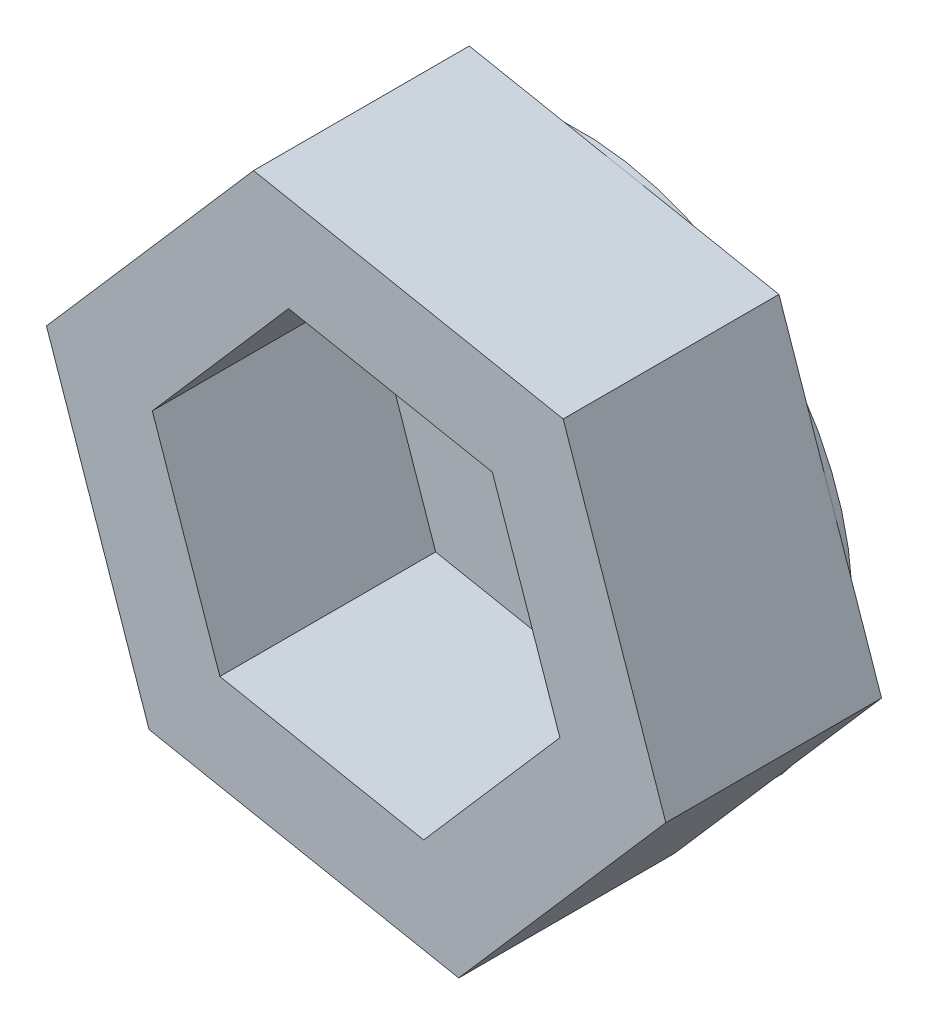
# Autodesk Inventor part: Part1
Saved by Autodesk Inventor 2014 SP1 (Build 180222100, 222)
## iProperties
Created: 2014-01-09
Part Number: Part1
Material: Generic
Document SubType Name: Modeling
Designer: Arpan
Density: 1 g/cm^3
Appearance: Default
Mass: 1.45957 g
Surface Area: 14.531 cm^2
Volume: 1.45957 cm^3
Author: Arpan
Autodesk Inventor part; units mm, degrees
ref_plane "YZ Plane" through (0, 0, 0) normal (1, 0, 0) x (0, 1, 0)
ref_plane "XZ Plane" through (0, 0, 0) normal (0, 1, 0) x (-1, 0, 0)
ref_plane "XY Plane" through (0, 0, 0) normal (0, 0, 1) x (1, 0, 0)
ref_plane "Work Plane1" through (500.3579, 35.9816, 443.1665) normal (0, 0, -1) x (0.6678, 0.7444, 0)
sketch "Sketch2" plane through (500.3579, 35.9816, 443.1665) normal (0, 0, -1) x (0.6678, 0.7444, 0)
  line L0 (3.7629, 6.2932) -> (-3.5686, 6.4054) projected
  line L1 (-3.5686, 6.4054) -> (-7.3315, 0.1122) projected
  line L2 (-7.3315, 0.1122) -> (-3.7629, -6.2932) projected
  line L3 (-3.7629, -6.2932) -> (3.5686, -6.4054) projected
  line L4 (3.5686, -6.4054) -> (7.3315, -0.1122) projected
  line L5 (7.3315, -0.1122) -> (3.7629, 6.2932) projected
  line L6 (-7.3315, 0.1122) -> (7.3315, -0.1122)
  line L7 (3.7629, 6.2932) -> (-3.7629, -6.2932)
  line L8 (-3.5686, 6.4054) -> (3.5686, -6.4054)
  line L9 (-3.5686, 6.4054) -> (-5.4229, 9.7337)
  line L10 (-5.4229, 9.7337) -> (5.7182, 9.5632)
  line L11 (5.7182, 9.5632) -> (11.141, -0.1705)
  line L12 (11.141, -0.1705) -> (5.4229, -9.7337)
  line L13 (5.4229, -9.7337) -> (-5.7182, -9.5632)
  line L14 (-5.7182, -9.5632) -> (-11.141, 0.1705)
  line L15 (-11.141, 0.1705) -> (-5.4229, 9.7337)
  point P0 (-360.9105, -348.4198)
  point P1 (0, 0)
  dimension "d0" = 3.81
  constraints: 20 end point, 3 parallel, 1 collinear, 1 midpoint, 13 other
  measures "d0" distance of L0.end L9.end
extrude "Extrusion1" add sketch "Sketch2" against normal blind 7.62
sketch "Sketch3" plane through (500.3579, 35.9816, 443.1665) normal (0, 0, -1) x (-0.7444, 0.6678, 0)
  line L0 (-6.2932, 3.7629) -> (0.1122, 7.3315) projected
  line L1 (0.1122, 7.3315) -> (6.4054, 3.5686) projected
  line L2 (6.4054, 3.5686) -> (6.2932, -3.7629) projected
  line L3 (6.2932, -3.7629) -> (-0.1122, -7.3315) projected
  line L4 (-0.1122, -7.3315) -> (-6.4054, -3.5686) projected
  line L5 (-6.4054, -3.5686) -> (-6.2932, 3.7629) projected
  line L6 (-9.7337, -5.4229) -> (-0.1705, -11.141) projected
  line L7 (-0.1705, -11.141) -> (9.5632, -5.7182) projected
  line L8 (9.5632, -5.7182) -> (9.7337, 5.4229) projected
  line L9 (9.7337, 5.4229) -> (0.1705, 11.141) projected
  line L10 (0.1705, 11.141) -> (-9.5632, 5.7182) projected
  line L11 (-9.5632, 5.7182) -> (-9.7337, -5.4229) projected
  point P0 (348.4198, -360.9105)
sketch "Sketch4" plane through (500.3579, 35.9816, 443.1665) normal (0, 0, -1) x (-0.7444, 0.6678, 0)
  circle A0 centre (0, 0) radius 9.6496
  circle A1 centre (0, 0) radius 3
  point P0 (348.4198, -360.9105)
  dimension "d3" = 6
  constraints: 2 centre point, 1 coincident, 3 other
  measures "d3" diameter of A1
extrude "Extrusion2" add sketch "Sketch4" along normal blind 0.25
body "Solid1"
